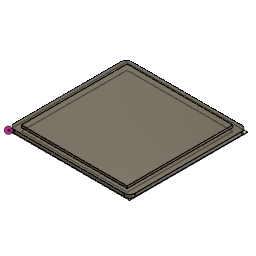
BOYES_BOX_LID v2 (Autodesk Fusion 360 design; units mm, degrees)
Autodesk Fusion 360 part; units mm, degrees
sketch "Sketch1" plane through (0, 0, 0) normal (0, 1, 0) x (1, 0, 0)
  line L0 (0, 0) -> (110, 0)
  line L1 (110, 0) -> (110, 107)
  line L2 (110, 107) -> (0, 107)
  line L3 (0, 107) -> (0, 0)
  line L4 (6.7, 5) -> (102.7, 5)
  line L5 (102.7, 5) -> (102.7, 101)
  line L6 (102.7, 101) -> (6.7, 101)
  line L7 (6.7, 101) -> (6.7, 5)
  dimension "d1" = 110
  dimension "d2" = 107
  dimension "d3" = 96
  dimension "d4" = 5
  dimension "d5" = 96
  dimension "d6" = 5.4
  dimension "d7" = 6.7
  dimension "d8" = 7.3
  measures "d1" distance of L0.start
  measures "d2" distance of L0.start
  measures "d3" distance of L5 L7
  measures "d4" distance of L0 L4
  measures "d5" distance of L4 L6
  measures "d6" distance of L2 L6
  measures "d7" distance of L3 L7
  measures "d8" distance of L1 L5
extrude "Extrude2" add sketch "Sketch1" along normal blind 3 makes body 1
extrude "Extrude1" add sketch "Sketch1" along normal blind 5 separate body contours L4 L5 L6 L7 makes body 2
fillet "Fillet1" radius 5 4 edges at (0, 1.5, 0) (110, 1.5, 0) (110, 1.5, -107) (0, 1.5, -107) on bodies 1
